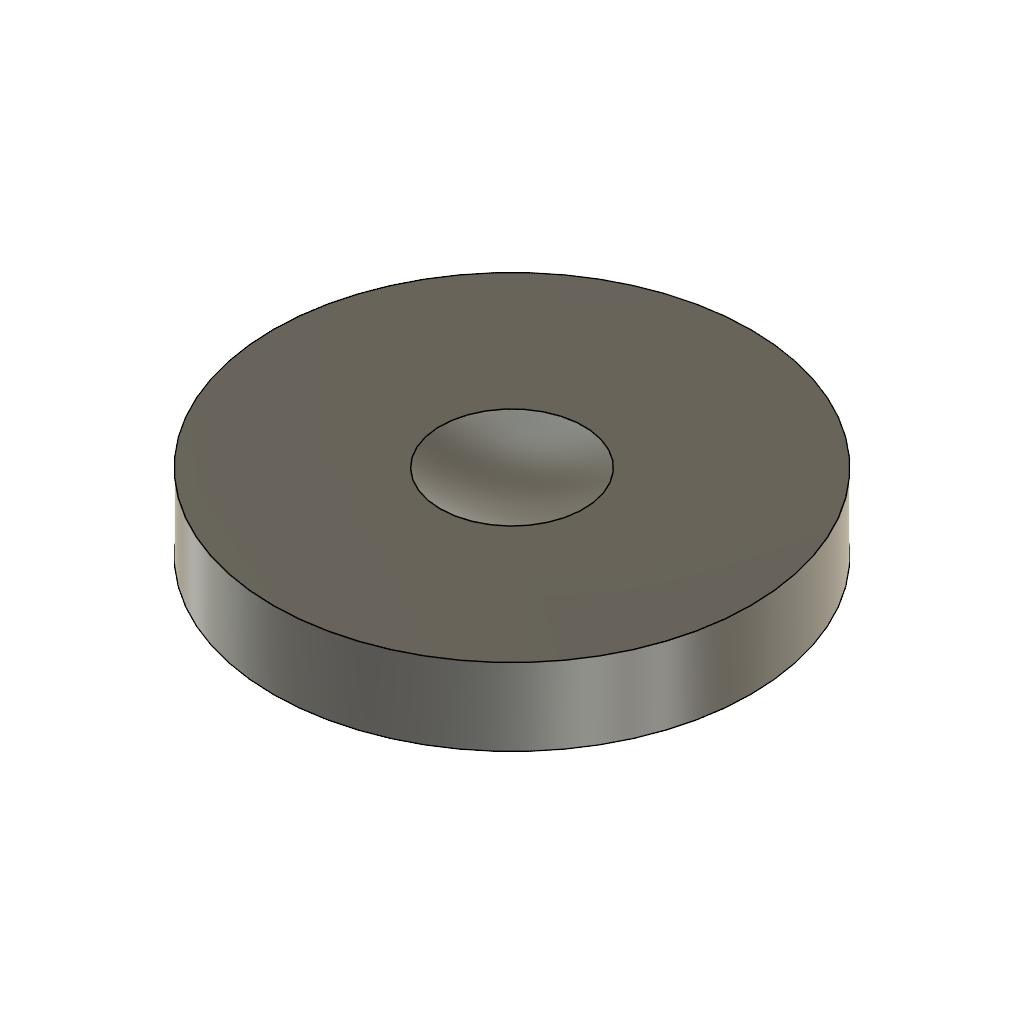
ITF_TB0301_platen_min_dimensions_v1 (Autodesk Fusion 360 design; units mm, degrees)
part number: 2026-09-29-11-46-47-461
Autodesk Fusion 360 part; units mm, degrees
sketch "Sketch1" plane through (0, 0, 0) normal (0, 0, 1) x (1, 0, 0)
  circle A0 centre (0, 0) radius 31
  dimension "d1" = 62
  constraint coincident A0.centre origin
  measures "d1" diameter of A0
extrude "Extrude1" add sketch "Sketch1" against normal blind 10
ref_plane "WorkPlane1" through (0, 0, -1.34) normal (0, 0, 1) x (1, 0, 0)
ref_plane "WorkPlane2" through (0, 0, 31.66) normal (0, 0, 1) x (1, 0, 0)
sketch "Sketch2" plane through (0, 0, 31.66) normal (0, 0, 1) x (1, 0, 0)
  circle A0 centre (0, 0) radius 33
  dimension "d8" = 66
  constraint coincident A0.centre origin
  measures "d8" diameter of A0
sphere "SpherePrimitive1" cut diameter 66 placed x (1, 0, 0) y (0, 1, 0) z (0, 0, 1) at (0, 0, 31.66)
named bodies: "ITF plate min. dimensions"
